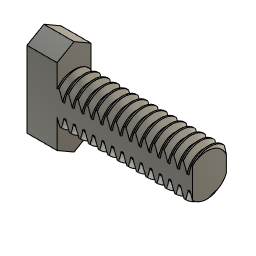
Printable 14-20 Bolt v1 (Autodesk Fusion 360 design; units mm, degrees)
Autodesk Fusion 360 part; units mm, degrees
sketch "Sketch1" plane through (0, 0, 0) normal (1, 0, 0) x (0, 1, 0)
  circle A0 centre (0, 0) radius 3.175
  dimension "d1" = 6.35
  constraint coincident A0.centre origin
  measures "d1" diameter of A0
extrude "Extrude1" add sketch "Sketch1" along normal blind 18
sketch "Sketch2" plane through (0, 0, 0) normal (-1, 0, 0) x (0, -1, 0)
  circle A0 centre (0, 0) radius 3.175
  line L0 (5.5, 3.1754) -> (0, 6.3509)
  line L1 (0, 6.3509) -> (-5.5, 3.1754)
  line L2 (-5.5, 3.1754) -> (-5.5, -3.1754)
  line L3 (-5.5, -3.1754) -> (0, -6.3509)
  line L4 (0, -6.3509) -> (5.5, -3.1754)
  line L5 (5.5, -3.1754) -> (5.5, 3.1754)
  dimension "d4" = 11
  constraint coincident A0.centre origin
  constraint vertical L5
  measures "d4" distance of L2 L5
extrude "Extrude2" add sketch "Sketch2" along normal blind 4 contours A0 | L0 L1 L2 L3 L4 L5
thread "Thread1" "ANSI Unified Screw Threads 0.25 1/4-20 UNC 3A" major diameter 6.2484 minor diameter 4.8387 pitch 1.27 angle 60 modelled right hand crest width 0.1965 on face at (12, 3.1711, -0.1583) crest through (-0.3175, 3.1242, 0)
sketch "Sketch3" plane through (-4, 0, 0) normal (-1, 0, 0) x (0, -1, 0)
  line L0 (5.5, -3.1754) -> (5.5, 3.1754)
  line L1 (5.5, 3.1754) -> (0, 6.3509)
  line L2 (0, 6.3509) -> (-5.5, 3.1754)
  line L3 (-5.5, 3.1754) -> (-5.5, -3.1754)
  line L4 (-5.5, -3.1754) -> (0, -6.3509)
  line L5 (0, -6.3509) -> (5.5, -3.1754)
  line L6 (0, 0) -> (0, 21) construction
  line L7 (0, 0) -> (0, -19) construction
  line L8 (2.25, 5.0518) -> (2.25, -5.0518)
  line L9 (-2.25, 5.0518) -> (-2.25, -5.0518)
  dimension "d7" = 2.25
  dimension "d8" = 2.25
  constraint coincident L6.start L7.start
  constraint parallel L0 L6
  constraint parallel L6 L7
  constraint coincident L1 L8.start
  constraint coincident L5 L8.end
  constraint parallel L6 L8
  constraint coincident L2 L9.start
  constraint coincident L4 L9.end
  constraint parallel L7 L9
  measures "d7" distance of L6.start L9
  measures "d8" distance of L6 L8
extrude "Extrude3" cut sketch "Sketch3" against normal through all contours L0 L1 L5 L8 | L2 L3 L4 L9
